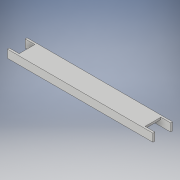
# Autodesk Inventor part: ArmProto2.2Assembly
Saved by Autodesk Inventor 2017 (Build 210142000, 142)
## iProperties
Created: 2017-10-04
Part Number: ArmProto2.2Assembly
Material: Generic
Document SubType Name: Modeling
Designer: User
Density: 1 g/cm^3
Appearance: Default
Author: User
Autodesk Inventor part; units mm, degrees
ref_plane "YZ Plane" through (0, 0, 0) normal (1, 0, 0) x (0, 1, 0)
ref_plane "XZ Plane" through (0, 0, 0) normal (0, 1, 0) x (-1, 0, 0)
ref_plane "XY Plane" through (0, 0, 0) normal (0, 0, 1) x (1, 0, 0)
sketch "Sketch1" plane through (0, 0, 0) normal (1, 0, 0) x (0, 1, 0)
  line L0 (0, 0) -> (25.4, 0)
  line L1 (25.4, 0) -> (25.4, -63.5)
  line L2 (25.4, -63.5) -> (0, -63.5)
  line L3 (0, -63.5) -> (0, 0)
  line L4 (0, -6.35) -> (19.05, -6.35)
  line L5 (19.05, -6.35) -> (19.05, -57.15)
  line L6 (19.05, -57.15) -> (0, -57.15)
  line L7 (0, -57.15) -> (0, -6.35)
  dimension "d0" = 25.4
  dimension "d1" = 63.5
  dimension "d2" = 50.8
  dimension "d3" = 19.05
  dimension "d4" = 6.35
  constraints: 16 end point, 4 parallel, 2 horizontal, 2 perpendicular, 1 point on line
  measures "d0" distance of L1.end L2.end
  measures "d1" distance of L0.end L1.end
  measures "d2" distance of L4.end L5.end
  measures "d3" distance of L5.end L6.end
  measures "d4" distance between parallel lines of L0 L4
extrude "Extrusion1" add sketch "Sketch1" along normal blind 469.9 contours L0 L1 L2 L3 L6 L5 L4
sketch "Sketch3" plane through (0, 25.4, 0) normal (0, 1, 0) x (1, 0, 0)
  line L0 (0, 63.5) -> (0, 0) projected
  line L1 (0, 0) -> (469.9, 0) projected
  line L2 (469.9, 63.5) -> (469.9, 0) projected
  line L3 (0, 63.5) -> (469.9, 63.5) projected
  line L4 (0, 6.35) -> (31.75, 6.35)
  line L5 (31.75, 6.35) -> (31.75, 57.15)
  line L6 (31.75, 57.15) -> (0, 57.15)
  line L7 (0, 57.15) -> (0, 6.35)
  line L8 (469.9, 57.15) -> (0, 57.15) projected
  line L9 (469.9, 6.35) -> (438.15, 6.35)
  line L10 (438.15, 6.35) -> (438.15, 57.15)
  line L11 (438.15, 57.15) -> (469.9, 57.15)
  line L12 (469.9, 57.15) -> (469.9, 6.35)
  dimension "d12" = 31.75
  dimension "d13" = 50.8
  dimension "d14" = 63.5
  dimension "d15" = 6.35
  dimension "d16" = 31.75
  constraints: 16 end point, 4 parallel, 3 point on line, 2 horizontal, 2 perpendicular
  measures "d12" distance of L6.end L5.end
  measures "d13" distance of L5.end L4.end
  measures "d14" distance of L0.start L0.end
  measures "d15" distance between parallel lines of L1 L4
  measures "d16" distance of L10.end L11.end
extrude "Extrusion2" cut sketch "Sketch3" against normal blind 6.35 contours L6 L5 L4 L0 | L2 L9 L10 L8
body "Solid1"
